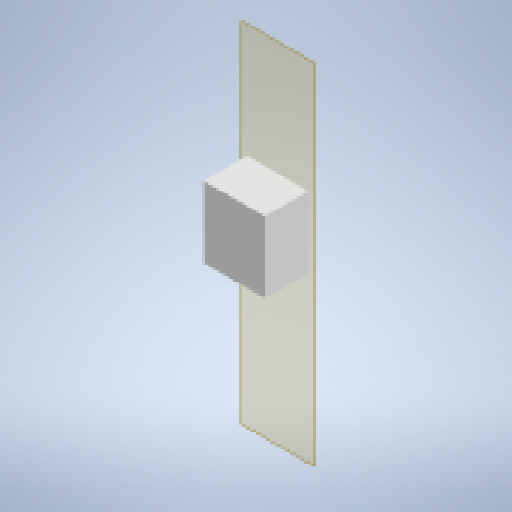
# Autodesk Inventor part: Battery1
Saved by Autodesk Inventor 2027.1 (Build 311270010, 270A)
## iProperties
Created: 2026-09-10
Part Number: Battery1
Material: Generic
Document SubType Name: Modeling
Designer: PWYNNE
Density: 1.8396 g/cm^3
Appearance: Default
Mass: 2680 g
Surface Area: 787.72 cm^2
Volume: 1456.84 cm^3
Author: PWYNNE
Autodesk Inventor part; units mm, degrees
ref_plane "YZ Plane" through (0, 0, 0) normal (1, 0, 0) x (0, 1, 0)
ref_plane "XZ Plane" through (0, 0, 0) normal (0, 1, 0) x (-1, 0, 0)
ref_plane "XY Plane" through (0, 0, 0) normal (0, 0, 1) x (1, 0, 0)
ref_plane "Work Plane1" through (0, 0, 0) normal (0, 0, 1) x (1, 0, 0)
sketch "Sketch1" plane through (0, 0, 0) normal (0, 0, 1) x (1, 0, 0)
  line L0 (-90, 284.1414) -> (-60, 284.1414) projected
  line L1 (-60, 284.1414) -> (-60, 404.1414) projected
  line L2 (-60, 404.1414) -> (-90, 404.1414) projected
  line L3 (-90, 404.1414) -> (-90, 284.1414) projected
  line L4 (-30, 414.1414) -> (-60, 414.1414) projected
  line L5 (-60, 414.1414) -> (-60, 284.1414) projected
  line L6 (-60, 284.1414) -> (-30, 284.1414) projected
  line L7 (-30, 284.1414) -> (-30, 414.1414) projected
  line L8 (-10, -149.0271) -> (-140, -149.0271) projected
  line L9 (-10, -149.0271) -> (-10, 350) projected
  spline S0 degree 3 poles (-55.3463, 478.2829) (-54.4199, 477.2402) (-53.5281, 476.1834) (-41.973, 461.9491) (-29.8681, 440.3891) (-13.701, 393.2059) (-10, 371.2252) (-10, 350) knots -13.956375 -13.956375 -13.956375 -13.956375 -13.398469 -13.398469 -6.367551 -6.367551 0 0 0 0 projected
  line L10 (-55.3463, 478.2829) -> (-94.6537, 478.2829) projected
  spline S1 degree 3 poles (-140, 350) (-140, 366.1219) (-137.8703, 382.0269) (-130.4211, 411.7266) (-125.3688, 425.7323) (-111.9139, 454.5302) (-103.4651, 468.0052) (-95.3677, 477.4713) (-95.011, 477.8807) (-94.6537, 478.2829) knots -5.300276 -5.300276 -5.300276 -5.300276 -3.93351 -3.93351 -2.695997 -2.695997 -1.209053 -1.209053 -1.140685 -1.140685 -1.140685 -1.140685 projected
  line L11 (-140, -149.0271) -> (-140, 350) projected
  line L12 (-10, 284.1414) -> (-140, 284.1414)
  line L13 (-140, 284.1414) -> (-140, -15.8586)
  line L14 (-140, -15.8586) -> (-10, -15.8586)
  line L15 (-10, -15.8586) -> (-10, 284.1414)
  point P0 (0, 0)
  point P1 (-10, -15.8586)
  dimension "d0" = 130
  dimension "d1" = 300
  constraints: 8 end point, 2 parallel, 1 horizontal, 1 perpendicular, 1 point on line
  measures "d0" distance of L14.end L13.end
  measures "d1" distance of L13.end L12.end
extrude "Extrusion1" add sketch "Sketch1" along normal blind 50 contours L0 L6 L12 L9 L14 L11
sketch "Sketch2" plane through (-140, 284.1414, 0) normal (0, 1, 0) x (1, 0, 0)
  line L0 (130, 0) -> (0, 0) projected
  line L1 (0, 0) -> (0, -50) projected
  line L2 (130, -50) -> (0, -50) projected
  line L3 (130, 0) -> (130, -50) projected
  line L4 (125.5, 0) -> (4.5, 0)
  line L5 (130, 0) -> (0, 0) projected
  line L6 (125.5, 0) -> (125.5, -86)
  line L7 (125.5, -86) -> (4.5, -86)
  line L8 (4.5, -86) -> (4.5, 0)
  line L9 (4.5, 0) -> (125.5, 0)
  line L10 (125.5, 0) -> (125.5, -86)
  line L11 (130, -50) -> (125.5, -50)
  line L12 (125.5, -50) -> (125.5, 0)
  line L13 (125.5, 0) -> (130, 0)
  line L14 (130, 0) -> (130, -50)
  line L15 (4.5, -50) -> (0, -50)
  line L16 (0, -50) -> (0, 0)
  line L17 (0, 0) -> (4.5, 0)
  line L18 (4.5, 0) -> (4.5, -50)
  point P0 (140, 0)
  point P1 (65, 0)
  dimension "d4" = 121
  dimension "d5" = 86
  constraints: 28 end point, 6 parallel, 4 perpendicular, 3 horizontal, 3 point on line, 2 midpoint
  measures "d4" distance of L4.start L4.end
  measures "d5" distance of L4.start L6.end
extrude "Extrusion2" cut sketch "Sketch2" against normal blind 300 contours L3 L2 L6 L0 | L8 L2 L1 L0
extrude "Extrusion3" add sketch "Sketch2" against normal blind 280 contours L6 L7 L8 L2
extrude "Extrusion4" cut sketch "Sketch2" against normal blind 300 contours L6 L2 L8 L0
extrude "Extrusion5" add sketch "Sketch2" against normal blind 280 contours L6 L2 L8 L0
sketch "Sketch3" plane through (-140, 4.1414, 0) normal (0, -1, 0) x (1, 0, 0)
  line L0 (125.5, 0) -> (125.5, 86) projected
  line L1 (125.5, 86) -> (4.5, 86) projected
  line L2 (4.5, 86) -> (4.5, 0) projected
  line L3 (4.5, 0) -> (125.5, 0) projected
  line L4 (4.5, 86) -> (125.5, 86)
  line L5 (125.5, 86) -> (125.5, 0)
  line L6 (125.5, 0) -> (4.5, 0)
  line L7 (4.5, 0) -> (4.5, 86)
  point P0 (140, 0)
  constraints: 8 end point, 2 parallel, 1 horizontal, 1 perpendicular
extrude "Extrusion6" cut sketch "Sketch3" against normal blind 140
body "Solid1"
